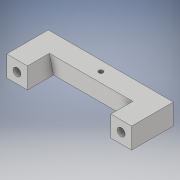
# Autodesk Inventor part: sliding piece for grabber
Saved by Autodesk Inventor 2019 (Build 230136000, 136)
## iProperties
Created: 2019-11-09
Part Number: sliding piece for grabber
Material: Generic
Document SubType Name: Modeling
Designer: User
Density: 1 g/cm^3
Appearance: Default
Author: User
Autodesk Inventor part; units mm, degrees
ref_plane "YZ Plane" through (0, 0, 0) normal (1, 0, 0) x (0, 1, 0)
ref_plane "XZ Plane" through (0, 0, 0) normal (0, 1, 0) x (-1, 0, 0)
ref_plane "XY Plane" through (0, 0, 0) normal (0, 0, 1) x (1, 0, 0)
sketch "Sketch1" plane through (0, 0, 0) normal (0, 1, 0) x (-1, 0, 0)
  line L0 (0, 0) -> (12.7, 0)
  line L1 (12.7, 0) -> (12.7, 25.4)
  line L2 (12.7, 25.4) -> (0, 25.4)
  line L3 (0, 25.4) -> (0, 0)
  line L4 (12.7, 0) -> (63.5, 0)
  line L5 (63.5, 0) -> (63.5, 9.525)
  line L6 (63.5, 9.525) -> (12.7, 9.525)
  line L7 (12.7, 9.525) -> (12.7, 0)
  line L8 (63.5, 0) -> (76.2, 0)
  line L9 (76.2, 0) -> (76.2, 25.4)
  line L10 (76.2, 25.4) -> (63.5, 25.4)
  line L11 (63.5, 25.4) -> (63.5, 0)
  dimension "d0" = 25.4
  dimension "d1" = 25.4
  dimension "d2" = 12.7
  dimension "d3" = 12.7
  dimension "d5" = 50.8
  dimension "d6" = 9.525
  constraints: 24 end point, 6 parallel, 3 horizontal, 3 perpendicular
  measures "d0" distance of L2.end L0.start
  measures "d1" distance of L8.end L9.end
  measures "d2" distance of L0.start L0.end
  measures "d3" distance of L4.end L8.end
  measures "d5" distance of L5.end L6.end
  measures "d6" distance between parallel lines of L6 L4
extrude "Extrusion1" add sketch "Sketch1" along normal blind 12.7
sketch "Sketch2" plane through (-63.5, 0, 25.4) normal (1, 0, 0) x (0, 0, -1)
  line L0 (15.875, 0) -> (15.875, 12.7) projected
  line L1 (15.875, 0) -> (13.335, 12.7)
  line L2 (0, 12.7) -> (15.875, 12.7) projected
  point P0 (25.4, 0)
  dimension "d9" = 2.54
  constraints: 2 end point, 1 point on line
  measures "d9" distance of L0.end L1.end
extrude "Extrusion2" add sketch "Sketch2" along normal blind 50.8
sketch "Sketch3" plane through (-76.2, 0, 25.4) normal (0, 0, 1) x (1, 0, 0)
  line L0 (0, 12.7) -> (12.7, 12.7) projected
  line L1 (0, 0) -> (0, 12.7) projected
  line L2 (63.5, 12.7) -> (76.2, 12.7) projected
  line L3 (76.2, 0) -> (76.2, 12.7) projected
  point P0 (6.35, 6.35)
  point P1 (69.85, 6.35)
  dimension "d12" = 12.7
  dimension "d13" = 12.7
  dimension "d14" = 6.35
  dimension "d15" = 6.35
  dimension "d16" = 12.7
  dimension "d17" = 12.7
  dimension "d18" = 6.35
  dimension "d19" = 6.35
  measures "d12" distance of L0.start L0.end
  measures "d13" distance of L1.start L0.start
  measures "d14" distance from line of L1 point (6.35, 6.35)
  measures "d15" distance from line of point (6.35, 6.35) L0
  measures "d16" distance of L2.start L2.end
  measures "d17" distance of L3.start L2.end
  measures "d18" distance from line of point (69.85, 6.35) L2
  measures "d19" distance from line of L3 point (69.85, 6.35)
hole "Hole1" at (-69.85, 6.35, 25.4) at (-6.35, 6.35, 25.4) direction (0, 0, -1) diameter 4.7625 end through all
sketch "Sketch4" plane through (0, 12.7, 0) normal (0, 1, 0) x (1, 0, 0)
  line L0 (0, 0) -> (-76.2, 0) projected
  line L1 (0, -25.4) -> (0, 0) projected
  line L2 (-12.7, -12.065) -> (-12.7, -25.4) projected
  point P0 (-38.1, -6.0325)
  dimension "d27" = 25.4
  dimension "d28" = 13.335
  dimension "d29" = 76.2
  dimension "d30" = 38.1
  dimension "d31" = 6.0325
  measures "d27" distance of L1.start L0.start
  measures "d28" distance of L2.start L2.end
  measures "d29" distance of L0.start L0.end
  measures "d30" distance from line of L1 point (-38.1, -6.033)
  measures "d31" distance from line of L0 point (-38.1, -6.033)
hole "Hole2" at (-38.1, 12.7, 6.0325) direction (0, -1, 0) diameter 2.6416 end through all thread size "6-32 UNC" class "2B" standard "ANSI Unified Screw Threads"
equation "\"d1\" = d0"
equation "\"d3\" = d2"
equation "\"d14\" = 0.5 * d12"
equation "\"d15\" = 0.5 * d13"
equation "\"d18\" = 0.5 * d17"
equation "\"d19\" = 0.5 * d16"
equation "\"d30\" = 0.5 * d29"
equation "\"d31\" = -0.5 * d28 + 0.5 * d27"
body "Solid1"
